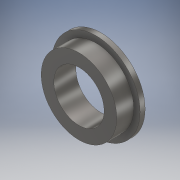
# Autodesk Inventor part: bear_f8_12_sa
Saved by Autodesk Inventor 2018 (Build 220112000, 112)
## iProperties
Created: 2018-06-20
Part Number: bear_f8_12_sa
Material: ステンレス鋼
Document SubType Name: Modeling
Designer: shun
Density: 8 g/cm^3
Appearance: 半つや出し
Author: shun
Autodesk Inventor part; units mm, degrees
ref_plane "YZ Plane" through (0, 0, 0) normal (1, 0, 0) x (0, 1, 0)
ref_plane "XZ Plane" through (0, 0, 0) normal (0, 1, 0) x (-1, 0, 0)
ref_plane "XY Plane" through (0, 0, 0) normal (0, 0, 1) x (1, 0, 0)
sketch "スケッチ1" plane through (0, 0, 0) normal (0, 0, 1) x (1, 0, 0)
  line L0 (4, 0) -> (4, -3.5)
  line L1 (4, 0) -> (7, 0)
  line L2 (7, 0) -> (7, -0.8)
  line L3 (7, -0.8) -> (6, -0.8)
  line L4 (6, -0.8) -> (6, -3.5)
  line L5 (6, -3.5) -> (4, -3.5)
  line L6 (0, -4.2) -> (0, 0.7) projected
  point P0 (0, 0)
  dimension "d2" = 3
  dimension "d3" = 0.8
  dimension "d4" = 1
  dimension "d5" = 4
  dimension "d6" = 3.5
  dimension "d7" = 3.5
  constraints: 12 end point, 4 perpendicular, 1 horizontal, 1 vertical
  measures "d2" distance of L0.start L1.end
  measures "d3" distance of L1.end L2.end
  measures "d4" distance of L2.end L3.end
  measures "d5" distance from line of point (0, 0) L0
  measures "d6" distance from line of point (0, 0) L5
  measures "d7" distance of L0.start L0.end
revolve "回転1" add sketch "スケッチ1" angle 360 about axis through (0, -10, 0) along (0, 1, 0)
